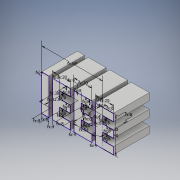
# Autodesk Inventor part: ieee
Saved by Autodesk Inventor 2017.2 (Build 212233000, 233)
## iProperties
Created: 2017-04-27
Part Number: ieee
Material: Generic
Document SubType Name: Modeling
Designer: visual15
Density: 1 g/cm^3
Appearance: Default
Author: visual15
Autodesk Inventor part; units mm, degrees
ref_plane "YZ Plane" through (0, 0, 0) normal (1, 0, 0) x (0, 1, 0)
ref_plane "XZ Plane" through (0, 0, 0) normal (0, 1, 0) x (-1, 0, 0)
ref_plane "XY Plane" through (0, 0, 0) normal (0, 0, 1) x (1, 0, 0)
sketch "Sketch1" plane through (0, 0, 0) normal (0, 0, 1) x (1, 0, 0)
  line L0 (0, 0) -> (68, 0) construction
  line L1 (68, 0) -> (68, 40) construction
  line L2 (68, 40) -> (0, 40) construction
  line L3 (0, 40) -> (0, 0) construction
  line L4 (0, 0) -> (8, 0)
  line L5 (8, 0) -> (8, 40)
  line L6 (8, 40) -> (0, 40)
  line L7 (0, 40) -> (0, 0)
  line L8 (12, 40) -> (12, 0)
  line L9 (12, 40) -> (32, 40)
  line L10 (32, 32) -> (20, 32)
  line L11 (20, 32) -> (20, 24)
  line L12 (20, 24) -> (32, 24)
  line L13 (32, 24) -> (32, 16)
  line L14 (32, 16) -> (20, 16)
  line L15 (20, 16) -> (20, 8)
  line L16 (32, 0) -> (12, 0)
  line L17 (32, 40) -> (32, 32)
  line L18 (20, 8) -> (32, 8)
  line L19 (32, 8) -> (32, 0)
  line L20 (36, 40) -> (36, 0)
  line L21 (36, 40) -> (56, 40)
  line L22 (56, 40) -> (56, 32)
  line L23 (44, 32) -> (56, 32)
  line L24 (44, 32) -> (44, 24)
  line L25 (56, 24) -> (44, 24)
  line L26 (56, 24) -> (56, 16)
  line L27 (56, 16) -> (44, 16)
  line L28 (44, 8) -> (44, 16)
  line L29 (44, 8) -> (56, 8)
  line L30 (56, 8) -> (56, 0)
  line L31 (56, 0) -> (36, 0)
  line L32 (60, 40) -> (60, 0)
  line L33 (60, 0) -> (80, 0)
  line L34 (80, 0) -> (80, 8)
  line L35 (68, 8) -> (80, 8)
  line L36 (68, 8) -> (68, 16)
  line L37 (68, 16) -> (80, 16)
  line L38 (80, 24) -> (68, 24)
  line L39 (68, 24) -> (80, 24)
  line L40 (80, 16) -> (80, 24)
  line L41 (68, 24) -> (68, 32)
  line L42 (80, 32) -> (68, 32)
  line L43 (80, 32) -> (80, 40)
  line L44 (60, 40) -> (80, 40)
  line L45 (0, 40) -> (0, 36)
  dimension "d0" = 68
  dimension "d1" = 40
  dimension "d2" = 8
  dimension "d3" = 4
  dimension "d4" = 8
  dimension "d5" = 8
  dimension "d6" = 8
  dimension "d7" = 8
  dimension "d8" = 20
  dimension "d9" = 8
  dimension "d10" = 20
  dimension "d11" = 8
  dimension "d12" = 8
  dimension "d15" = 8
  dimension "d16" = 4
  dimension "d17" = 8
  dimension "d18" = 8
  dimension "d19" = 8
  dimension "d20" = 8
  dimension "d21" = 8
  dimension "d22" = 8
  dimension "d23" = 4
  dimension "d24" = 20
  dimension "d25" = 8
  dimension "d34" = 4
  constraints: 90 end point, 20 point on line, 19 perpendicular, 6 horizontal, 6 vertical, 5 collinear, 4 parallel, 10 other
  measures "d0" distance of L3.start L1.end
  measures "d1" distance of L1.end L0.end
  measures "d2" distance between parallel lines of L3 L5
  measures "d3" distance between parallel lines of L5 L8
  measures "d4" distance of L9.end L10.start
  measures "d5" distance of L10.end L11.end
  measures "d6" distance of L12.end L13.end
  measures "d7" distance of L14.end L15.end
  measures "d8" distance between parallel lines of L8 L17
  measures "d9" distance between parallel lines of L8 L11
  measures "d10" distance between parallel lines of L20 L22
  measures "d11" distance between parallel lines of L24 L20
  measures "d12" distance of L21.end L22.end
  measures "d15" distance between parallel lines of L29 L27
  measures "d16" distance between parallel lines of L19 L20
  measures "d17" distance between parallel lines of L27 L25
  measures "d18" distance between parallel lines of L25 L23
  measures "d20" distance between parallel lines of L39 L42
  measures "d21" distance between parallel lines of L37 L39
  measures "d22" distance between parallel lines of L35 L37
  measures "d23" distance between parallel lines of L30 L32
  measures "d24" distance between parallel lines of L32 L43
  measures "d25" distance between parallel lines of L32 L41
  measures "d34" distance of L45.end L3.start
extrude "Extrusion1" add sketch "Sketch1" against normal blind 40
sketch "Sketch4" plane through (0, 0, 0) normal (0, -1, 0) x (1, 0, 0)
  line L0 (8, -40) -> (0, -40) construction
  line L1 (0, -32) -> (0, -10)
  line L2 (0, 0) -> (0, -40) construction
  line L3 (0, -10) -> (8, -10)
  line L4 (8, -10) -> (8, -32.5)
  line L5 (8, -32.5) -> (16, -32.5)
  line L6 (16, -32.5) -> (16, -10)
  line L7 (24, -10) -> (16, -10)
  line L8 (24, -10) -> (24, -32)
  line L9 (20, 0) -> (20, -40) construction
  line L10 (8, -40) -> (16, -40)
  line L11 (12, -40) -> (32, -40) construction
  arc A0 (0, -32) -> (8, -40) centre (8, -32) ccw
  arc A1 (16, -40) -> (24, -32) centre (16, -32) ccw
  line L12 (28, -10) -> (28, -40)
  line L13 (36, 0) -> (36, -40) construction
  line L14 (28, -10) -> (52, -10)
  line L15 (36, -18) -> (44, -18)
  line L16 (44, -18) -> (44, -26)
  line L17 (44, -26) -> (36, -26)
  line L18 (36, -26) -> (36, -18)
  line L19 (56, 0) -> (56, -40) construction
  line L20 (24, -10) -> (24, -40) construction
  line L21 (44, 0) -> (44, -40) construction
  line L22 (52, -10) -> (52, -30)
  line L23 (52, -30) -> (49.1514, -30)
  line L24 (49.1514, -30) -> (53.3027, -40)
  line L25 (53.3027, -40) -> (45.3027, -40)
  line L26 (45.3027, -40) -> (41.1514, -30)
  line L27 (41.1514, -30) -> (36, -30)
  line L28 (36, -30) -> (36, -40)
  line L29 (36, -40) -> (28, -40)
  dimension "d36" = 8
  dimension "d37" = 8
  dimension "d38" = 8
  dimension "d39" = 22.5
  dimension "d40" = 30
  dimension "d41" = 8
  dimension "d42" = 4
  dimension "d46" = 24
  dimension "d47" = 30
  dimension "d48" = 8
  dimension "d49" = 8
  dimension "d50" = 8
  dimension "d51" = 8
  dimension "d52" = 8
  dimension "d53" = 8
  dimension "d54" = 4
  dimension "d55" = 30
  constraints: 46 end point, 8 point on line, 7 perpendicular, 5 parallel, 4 point on circle, 4 tangent, 3 collinear, 3 vertical, 2 centre point, 2 horizontal, 1 equal radius
  measures "d36" distance of L1.end L3.end
  measures "d37" distance of L7.start L6.end
  measures "d38" distance of L4.end L5.end
  measures "d39" distance between parallel lines of L3 L5
  measures "d40" distance between parallel lines of L0 L3
  measures "d41" radius of A0
  measures "d42" distance between parallel lines of L8 L12
  measures "d46" distance of L12.start L14.end
  measures "d47" distance of L12.start L12.end
  measures "d48" distance between parallel lines of L14 L15
  measures "d49" distance between parallel lines of L12 L18
  measures "d50" distance of L16.end L17.end
  measures "d51" distance of L15.end L16.end
  measures "d52" distance of L28.end L12.end
  measures "d53" distance of L24.end L25.end
  measures "d54" distance between parallel lines of L17 L27
  measures "d55" distance between parallel lines of L25 L14
equation "\"d0\" = 1.7 * d1"
equation "\"d2\" = 0.2 * d1"
equation "\"d3\" = 0.5 * d2"
equation "\"d4\" = 0.2 * d1"
equation "\"d5\" = d4"
equation "\"d6\" = d5"
equation "\"d7\" = d6"
equation "\"d8\" = 2.5 * d2"
equation "\"d9\" = d2"
equation "\"d10\" = d8"
equation "\"d11\" = d9"
equation "\"d12\" = d4"
equation "\"d15\" = d4"
equation "\"d16\" = d3"
equation "\"d18\" = d4"
equation "\"d19\" = d4"
equation "\"d20\" = d4"
equation "\"d21\" = d4"
equation "\"d22\" = d4"
equation "\"d23\" = d3"
equation "\"d24\" = d8"
equation "\"d25\" = d9"
equation "\"d34\" = 0.5 * d2"
equation "\"d36\" = d2"
equation "\"d37\" = d2"
equation "\"d38\" = d2"
equation "\"d39\" = 0.75 * d40"
equation "\"d40\" = 0.75 * d1"
equation "\"d41\" = d2"
equation "\"d42\" = 0.5 * d2"
equation "\"d46\" = 3 * d2"
equation "\"d47\" = d40"
equation "\"d48\" = d2"
equation "\"d49\" = d2"
equation "\"d50\" = d2"
equation "\"d51\" = d2"
equation "\"d52\" = d2"
equation "\"d53\" = d2"
equation "\"d54\" = 0.5 * d2"
equation "\"d55\" = d47"
body "Solid1"
